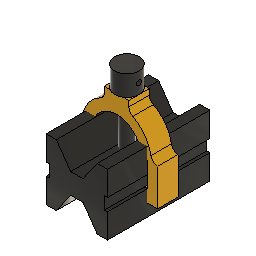
Advance Design 2 v1 (Autodesk Fusion 360 design; units mm, degrees)
Autodesk Fusion 360 part; units mm, degrees
sketch "Sketch1" plane through (0, 0, 0) normal (0, 1, 0) x (1, 0, 0) in component "Base "
  line L0 (270, 60) -> (300, 60)
  line L1 (300, -60) -> (270, -60)
  line L2 (270, -60) -> (270, 60)
  line L3 (0, 0) -> (0, 100) construction
  line L4 (270, 0) -> (300, 0) construction
  line L5 (200, 300) -> (60, 100)
  line L6 (60, 100) -> (0, 100)
  line L7 (-60, 100) -> (0, 100)
  line L8 (-200, 300) -> (-60, 100)
  line L9 (-60, -100) -> (0, -100)
  line L10 (-200, -300) -> (-60, -100)
  line L11 (60, -100) -> (0, -100)
  line L12 (200, -300) -> (60, -100)
  line L13 (-270, 60) -> (-300, 60)
  line L14 (-270, -60) -> (-270, 60)
  line L15 (-300, -60) -> (-270, -60)
  line L16 (300, -300) -> (200, -300)
  line L17 (-200, -300) -> (-300, -300)
  line L18 (300, 300) -> (300, 60)
  line L19 (300, -60) -> (300, -300)
  line L20 (-300, 300) -> (-200, 300)
  line L21 (200, 300) -> (300, 300)
  line L22 (-300, -300) -> (-300, -60)
  line L23 (-300, 60) -> (-300, 300)
  dimension "d1" = 600
  dimension "d2" = 600
  dimension "d5" = 100
  dimension "d6" = 200
  dimension "d7" = 120
  constraint horizontal L20
  constraint perpendicular L18 L20
  constraint parallel L16 L20
  constraint parallel L18 L22
  constraint coincident L3.start origin
  constraint horizontal L0
  constraint parallel L0 L1
  constraint perpendicular L3 L20
  constraint perpendicular L4 L18
  constraint coincident L5.start L20
  constraint perpendicular L3 L6
  constraint symmetric L3 L5.start L8.start
  constraint symmetric L3 L5.end L7.start
  constraint symmetric L4 L5.start L12.start
  constraint symmetric L4 L5.end L11.start
  constraint symmetric L4 L3.end L9.end
  constraint symmetric L4 L7.start L9.start
  constraint symmetric L4 L8.start L10.start
  constraint symmetric L0.start L3 L13.start
  constraint symmetric L1.end L3 L14.start
  constraint collinear L16 L17
  constraint collinear L18 L19
  constraint collinear L20 L21
  constraint coincident L13.end L22
  constraint collinear L22 L23
  constraint coincident L2 L4.start
  measures "d1" distance of L16.start L17.end
  measures "d2" distance of L18.start L16.start
  measures "d5" distance of L20.start L8.start
  measures "d6" distance of L7 L20
  measures "d7" distance of L5.end L7.start
extrude "Extrude1" add sketch "Sketch1" along normal mid plane 1000 makes body 1 in component "Base "
sketch "Sketch1 (2)" plane through (0, 0, 0) normal (0, 1, 0) x (1, 0, 0) in component "Slider"
  line L0 (-60, -100) -> (-200, -300)
  line L1 (-200, -300) -> (-300, -300)
  line L2 (-300, -300) -> (-300, -60)
  line L3 (-300, -60) -> (-270, -60)
  line L4 (-270, -60) -> (-270, 60)
  line L5 (-270, 60) -> (-300, 60)
  line L6 (-300, 60) -> (-300, 300)
  line L7 (-300, 300) -> (-200, 300)
  line L8 (-200, 300) -> (-60, 100)
  line L9 (-60, 100) -> (60, 100)
  line L10 (60, 100) -> (200, 300)
  line L11 (200, 300) -> (300, 300)
  line L12 (300, 300) -> (300, 60)
  line L13 (300, 60) -> (270, 60)
  line L14 (270, 60) -> (270, -60)
  line L15 (270, -60) -> (300, -60)
  line L16 (300, -60) -> (300, -300)
  line L17 (300, -300) -> (200, -300)
  line L18 (200, -300) -> (60, -100)
  line L19 (60, -100) -> (-60, -100)
  line L20 (300, 60) -> (400, 60)
  line L21 (400, 60) -> (400, -300)
  arc A0 (-240, -300) -> (240, -300) centre (0, -300) ccw
  arc A1 (-340, -300) -> (340, -300) centre (0, -300) ccw
  line L22 (340, -300) -> (400, -300)
  line L23 (0, 0) -> (0, -900) construction
  line L24 (0, 0) -> (800, 0) construction
  line L25 (-300, 60) -> (-400, 60)
  line L26 (-340, -300) -> (-400, -300)
  line L27 (-400, 60) -> (-400, -300)
  line L28 (120, -618.1195) -> (-120, -618.1195)
  line L29 (-120, -618.1195) -> (-120, -718.1195)
  line L30 (-120, -718.1195) -> (120, -718.1195)
  line L31 (120, -718.1195) -> (120, -618.1195)
  line L32 (120, -618.1195) -> (-120, -718.1195) construction
  line L33 (-120, -618.1195) -> (120, -718.1195) construction
  point P0 (0, -668.1195)
  dimension "d10" = 100
  dimension "d11" = 240
  dimension "d12" = 340
  dimension "d13" = 100
  dimension "d14" = 240
  constraint coincident L12.end L13.start
  constraint perpendicular L12 L20
  constraint perpendicular L20 L21
  constraint coincident A0.centre A1.centre
  constraint perpendicular L21 L22
  constraint coincident L23.start L24.start
  constraint parallel L16 L23
  constraint perpendicular L14 L24
  constraint symmetric L12.end L23 L5.end
  constraint symmetric L20.end L23 L25.end
  constraint symmetric L21.end L23 L26.end
  constraint symmetric A1.end L23 A1.start
  constraint horizontal L28
  constraint perpendicular L28 L29
  constraint parallel L28 L30
  constraint parallel L29 L31
  constraint coincident L32 P0
  constraint coincident L33 P0
  constraint coincident A1 L28.start
  constraint coincident L23 P0
  measures "d10" distance of L12.end L20.end
  measures "d11" radius of A0
  measures "d12" radius of A1
  measures "d13" distance of L28.end L29.end
  measures "d14" distance of L29.end L30.end
extrude "Extrude1'" add sketch "Sketch1 (2)" along normal mid plane 200 separate body contours L1 L2 L3 L4 L5 L13 L14 L15 L16 L17 L20 L21 A0 A1 L22 L25 L26 L27 L28 | A1 L28 | A1 L29 L30 L31 makes body 2 in component "Slider"
hole "Hole1" at (0, 0, 718.1195) direction (0, 0, -1) diameter 120 end through all bodies 2 in component "Slider"
fillet "Fillet1" radius 70 4 edges at (120, 0, 618.1195) (340, 0, 300) (-340, 0, 300) (-120, 0, 618.1195) on bodies 2 in component "Slider"
cylinder "CylinderPrimitive1" add diameter 120 height 600 placed x (1, 0, 0) y (0, 1, 0) z (0, 0, 1) at (0, 0, 718.1195) separate body makes body 3 in component "Pin"
cylinder "CylinderPrimitive2" add diameter 240 height 200 placed x (1, 0, 0) y (0, 1, 0) z (0, 0, 1) at (0, 0, 1318.1195) bodies 3 in component "Pin"
hole "Hole1'" at (120, 0, 1418.1195) direction (-1, 0, 0) diameter 50 end through all bodies 3 in component "Pin"
component "Base " placed x (1, 0, 0) y (0, 1, 0) z (0, 0, 1) at (0, 0, 0)
component "Slider" placed x (1, 0, 0) y (0, 1, 0) z (0, 0, 1) at (0, 500, -120)
component "Pin" placed x (1, 0, 0) y (0, 1, 0) z (0, 0, 1) at (0, 500, -720)
